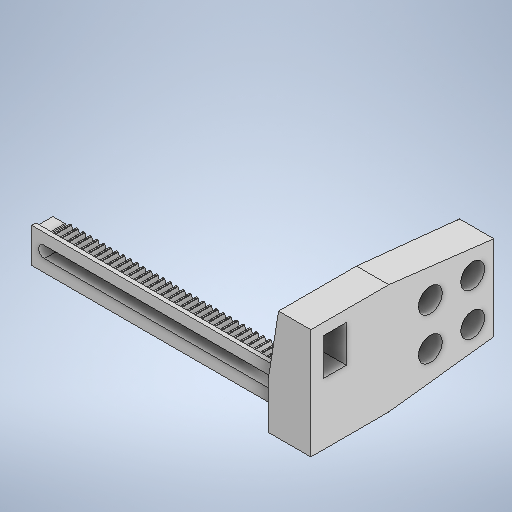
# Autodesk Inventor part: Gripper_Finger
Saved by Autodesk Inventor 2025.1 (Build 291241000, 241)
## iProperties
Created: 2024-08-01
Part Number: Gripper_Finger
Material: Generic
Document SubType Name: Modeling
Designer: leonh
Density: 1 g/cm^3
Appearance: Default
Author: leonh
Autodesk Inventor part; units mm, degrees
(part 1 of 3)
ref_plane "YZ Plane" through (0, 0, 0) normal (1, 0, 0) x (0, 1, 0)
ref_plane "XZ Plane" through (0, 0, 0) normal (0, 1, 0) x (-1, 0, 0)
sketch "Sketch1" plane through (0, 0, 0) normal (0, 0, 1) x (1, 0, 0)
  line L0 (-2.8751, 1.4125) -> (2.9873, 1.4125) construction
  line L1 (-2.8751, 0.2875) -> (2.9873, 0.2875) construction
  line L2 (-2.4544, 1.4586) -> (-2.4544, -0.4067) construction
  line L3 (-2.0617, 1.4586) -> (-2.0617, -0.3717) construction
  line L4 (-1.669, 1.4586) -> (-1.669, -0.4628) construction
  line L5 (-1.2763, 1.4586) -> (-1.2763, -0.4628) construction
  line L6 (-0.8836, 1.4586) -> (-0.8836, -0.5795) construction
  line L7 (-2.8751, 0.9125) -> (-2.5944, 0.9125) construction
  line L8 (-1.8366, 0.452) -> (-1.669, 0.9125)
  line L9 (-1.669, 0.9125) -> (-1.5109, 1.3467)
  line L10 (-1.0416, 1.3467) -> (-0.8836, 0.9125)
  line L11 (-2.2868, 0.452) -> (-2.4065, 0.7809)
  line L12 (-1.417, 1.4125) -> (-1.0656, 1.4125) construction
  line L13 (-2.0518, 0.2875) -> (-2.0715, 0.2875)
  line L14 (-1.487, 1.4125) -> (-1.1356, 1.4125)
  arc A0 (-2.2868, 0.452) -> (-2.0518, 0.2875) centre (-2.0518, 0.5375) ccw
  arc A1 (-2.0715, 0.2875) -> (-1.8366, 0.452) centre (-2.0715, 0.5375) ccw
  arc A2 (-1.417, 1.4125) -> (-1.5109, 1.3467) centre (-1.417, 1.3125) ccw
  arc A3 (-1.0416, 1.3467) -> (-1.1356, 1.4125) centre (-1.1356, 1.3125) ccw
  arc A4 (0.5292, 1.3467) -> (0.4352, 1.4125) centre (0.4352, 1.3125) ccw
  line L15 (0.1538, 1.4125) -> (0.5052, 1.4125) construction
  arc A5 (0.1538, 1.4125) -> (0.0599, 1.3467) centre (0.1538, 1.3125) ccw
  line L16 (-0.0982, 0.9125) -> (0.0599, 1.3467)
  line L17 (0.0838, 1.4125) -> (0.4352, 1.4125)
  line L18 (-0.2658, 0.452) -> (-0.0982, 0.9125)
  arc A6 (-0.5007, 0.2875) -> (-0.2658, 0.452) centre (-0.5007, 0.5375) ccw
  line L19 (-0.481, 0.2875) -> (-0.5007, 0.2875)
  arc A7 (-0.716, 0.452) -> (-0.481, 0.2875) centre (-0.481, 0.5375) ccw
  line L20 (-0.716, 0.452) -> (-0.8836, 0.9125)
  line L21 (0.5292, 1.3467) -> (0.6872, 0.9125)
  arc A8 (2.1, 1.3467) -> (2.006, 1.4125) centre (2.006, 1.3125) ccw
  line L22 (1.7246, 1.4125) -> (2.076, 1.4125) construction
  arc A9 (1.7246, 1.4125) -> (1.6307, 1.3467) centre (1.7246, 1.3125) ccw
  line L23 (1.4726, 0.9125) -> (1.6307, 1.3467)
  line L24 (1.6546, 1.4125) -> (2.006, 1.4125)
  line L25 (1.305, 0.452) -> (1.4726, 0.9125)
  arc A10 (1.0701, 0.2875) -> (1.305, 0.452) centre (1.0701, 0.5375) ccw
  line L26 (1.0898, 0.2875) -> (1.0701, 0.2875)
  arc A11 (0.8548, 0.452) -> (1.0898, 0.2875) centre (1.0898, 0.5375) ccw
  line L27 (0.8548, 0.452) -> (0.6872, 0.9125)
  line L28 (2.1, 1.3467) -> (2.258, 0.9125)
  arc A12 (3.6708, 1.3467) -> (3.5768, 1.4125) centre (3.5768, 1.3125) ccw
  line L29 (3.2954, 1.4125) -> (3.6468, 1.4125) construction
  arc A13 (3.2954, 1.4125) -> (3.2015, 1.3467) centre (3.2954, 1.3125) ccw
  line L30 (3.0434, 0.9125) -> (3.2015, 1.3467)
  line L31 (3.2254, 1.4125) -> (3.5768, 1.4125)
  line L32 (2.8758, 0.452) -> (3.0434, 0.9125)
  arc A14 (2.6409, 0.2875) -> (2.8758, 0.452) centre (2.6409, 0.5375) ccw
  line L33 (2.6606, 0.2875) -> (2.6409, 0.2875)
  arc A15 (2.4256, 0.452) -> (2.6606, 0.2875) centre (2.6606, 0.5375) ccw
  line L34 (2.4256, 0.452) -> (2.258, 0.9125)
  line L35 (3.6708, 1.3467) -> (3.8288, 0.9125)
  arc A16 (5.2416, 1.3467) -> (5.1476, 1.4125) centre (5.1476, 1.3125) ccw
  line L36 (4.8662, 1.4125) -> (5.2176, 1.4125) construction
  arc A17 (4.8662, 1.4125) -> (4.7723, 1.3467) centre (4.8662, 1.3125) ccw
  line L37 (4.6142, 0.9125) -> (4.7723, 1.3467)
  line L38 (4.7962, 1.4125) -> (5.1476, 1.4125)
  line L39 (4.4466, 0.452) -> (4.6142, 0.9125)
  arc A18 (4.2117, 0.2875) -> (4.4466, 0.452) centre (4.2117, 0.5375) ccw
  line L40 (4.2313, 0.2875) -> (4.2117, 0.2875)
  arc A19 (3.9964, 0.452) -> (4.2313, 0.2875) centre (4.2313, 0.5375) ccw
  line L41 (3.9964, 0.452) -> (3.8288, 0.9125)
  line L42 (5.2416, 1.3467) -> (5.3996, 0.9125)
  arc A20 (6.8124, 1.3467) -> (6.7184, 1.4125) centre (6.7184, 1.3125) ccw
  line L43 (6.437, 1.4125) -> (6.7884, 1.4125) construction
  arc A21 (6.437, 1.4125) -> (6.343, 1.3467) centre (6.437, 1.3125) ccw
  line L44 (6.185, 0.9125) -> (6.343, 1.3467)
  line L45 (6.367, 1.4125) -> (6.7184, 1.4125)
  line L46 (6.0174, 0.452) -> (6.185, 0.9125)
  arc A22 (5.7825, 0.2875) -> (6.0174, 0.452) centre (5.7825, 0.5375) ccw
  line L47 (5.8021, 0.2875) -> (5.7825, 0.2875)
  arc A23 (5.5672, 0.452) -> (5.8021, 0.2875) centre (5.8021, 0.5375) ccw
  line L48 (5.5672, 0.452) -> (5.3996, 0.9125)
  line L49 (6.8124, 1.3467) -> (6.9704, 0.9125)
  arc A24 (8.3832, 1.3467) -> (8.2892, 1.4125) centre (8.2892, 1.3125) ccw
  line L50 (8.0078, 1.4125) -> (8.3592, 1.4125) construction
  arc A25 (8.0078, 1.4125) -> (7.9138, 1.3467) centre (8.0078, 1.3125) ccw
  line L51 (7.7558, 0.9125) -> (7.9138, 1.3467)
  line L52 (7.9378, 1.4125) -> (8.2892, 1.4125)
  line L53 (7.5882, 0.452) -> (7.7558, 0.9125)
  arc A26 (7.3533, 0.2875) -> (7.5882, 0.452) centre (7.3533, 0.5375) ccw
  line L54 (7.3729, 0.2875) -> (7.3533, 0.2875)
  arc A27 (7.138, 0.452) -> (7.3729, 0.2875) centre (7.3729, 0.5375) ccw
  line L55 (7.138, 0.452) -> (6.9704, 0.9125)
  line L56 (8.3832, 1.3467) -> (8.5412, 0.9125)
  arc A28 (9.954, 1.3467) -> (9.86, 1.4125) centre (9.86, 1.3125) ccw
  line L57 (9.5786, 1.4125) -> (9.93, 1.4125) construction
  arc A29 (9.5786, 1.4125) -> (9.4846, 1.3467) centre (9.5786, 1.3125) ccw
  line L58 (9.3266, 0.9125) -> (9.4846, 1.3467)
  line L59 (9.5086, 1.4125) -> (9.86, 1.4125)
  line L60 (9.159, 0.452) -> (9.3266, 0.9125)
  arc A30 (8.9241, 0.2875) -> (9.159, 0.452) centre (8.9241, 0.5375) ccw
  line L61 (8.9437, 0.2875) -> (8.9241, 0.2875)
  arc A31 (8.7088, 0.452) -> (8.9437, 0.2875) centre (8.9437, 0.5375) ccw
  line L62 (8.7088, 0.452) -> (8.5412, 0.9125)
  line L63 (9.954, 1.3467) -> (10.112, 0.9125)
  arc A32 (11.5248, 1.3467) -> (11.4308, 1.4125) centre (11.4308, 1.3125) ccw
  line L64 (11.1494, 1.4125) -> (11.5008, 1.4125) construction
  arc A33 (11.1494, 1.4125) -> (11.0554, 1.3467) centre (11.1494, 1.3125) ccw
  line L65 (10.8974, 0.9125) -> (11.0554, 1.3467)
  line L66 (11.0794, 1.4125) -> (11.4308, 1.4125)
  line L67 (10.7298, 0.452) -> (10.8974, 0.9125)
  arc A34 (10.4949, 0.2875) -> (10.7298, 0.452) centre (10.4949, 0.5375) ccw
  line L68 (10.5145, 0.2875) -> (10.4949, 0.2875)
  arc A35 (10.2796, 0.452) -> (10.5145, 0.2875) centre (10.5145, 0.5375) ccw
  line L69 (10.2796, 0.452) -> (10.112, 0.9125)
  line L70 (11.5248, 1.3467) -> (11.6828, 0.9125)
  arc A36 (13.0956, 1.3467) -> (13.0016, 1.4125) centre (13.0016, 1.3125) ccw
  line L71 (12.7202, 1.4125) -> (13.0716, 1.4125) construction
  arc A37 (12.7202, 1.4125) -> (12.6262, 1.3467) centre (12.7202, 1.3125) ccw
  line L72 (12.4682, 0.9125) -> (12.6262, 1.3467)
  line L73 (12.6502, 1.4125) -> (13.0016, 1.4125)
  line L74 (12.3006, 0.452) -> (12.4682, 0.9125)
  arc A38 (12.0657, 0.2875) -> (12.3006, 0.452) centre (12.0657, 0.5375) ccw
  line L75 (12.0853, 0.2875) -> (12.0657, 0.2875)
  arc A39 (11.8504, 0.452) -> (12.0853, 0.2875) centre (12.0853, 0.5375) ccw
  line L76 (11.8504, 0.452) -> (11.6828, 0.9125)
  line L77 (13.0956, 1.3467) -> (13.2536, 0.9125)
  arc A40 (14.6664, 1.3467) -> (14.5724, 1.4125) centre (14.5724, 1.3125) ccw
  line L78 (14.291, 1.4125) -> (14.6424, 1.4125) construction
  arc A41 (14.291, 1.4125) -> (14.197, 1.3467) centre (14.291, 1.3125) ccw
  line L79 (14.039, 0.9125) -> (14.197, 1.3467)
  line L80 (14.221, 1.4125) -> (14.5724, 1.4125)
  line L81 (13.8714, 0.452) -> (14.039, 0.9125)
  arc A42 (13.6365, 0.2875) -> (13.8714, 0.452) centre (13.6365, 0.5375) ccw
  line L82 (13.6561, 0.2875) -> (13.6365, 0.2875)
  arc A43 (13.4212, 0.452) -> (13.6561, 0.2875) centre (13.6561, 0.5375) ccw
  line L83 (13.4212, 0.452) -> (13.2536, 0.9125)
  line L84 (14.6664, 1.3467) -> (14.8244, 0.9125)
  arc A44 (16.2372, 1.3467) -> (16.1432, 1.4125) centre (16.1432, 1.3125) ccw
  line L85 (15.8618, 1.4125) -> (16.2132, 1.4125) construction
  arc A45 (15.8618, 1.4125) -> (15.7678, 1.3467) centre (15.8618, 1.3125) ccw
  line L86 (15.6098, 0.9125) -> (15.7678, 1.3467)
  line L87 (15.7918, 1.4125) -> (16.1432, 1.4125)
  line L88 (15.4422, 0.452) -> (15.6098, 0.9125)
  arc A46 (15.2073, 0.2875) -> (15.4422, 0.452) centre (15.2073, 0.5375) ccw
  line L89 (15.2269, 0.2875) -> (15.2073, 0.2875)
  arc A47 (14.992, 0.452) -> (15.2269, 0.2875) centre (15.2269, 0.5375) ccw
  line L90 (14.992, 0.452) -> (14.8244, 0.9125)
  line L91 (16.2372, 1.3467) -> (16.3952, 0.9125)
  arc A48 (17.8079, 1.3467) -> (17.714, 1.4125) centre (17.714, 1.3125) ccw
  line L92 (17.4326, 1.4125) -> (17.784, 1.4125) construction
  arc A49 (17.4326, 1.4125) -> (17.3386, 1.3467) centre (17.4326, 1.3125) ccw
  line L93 (17.1806, 0.9125) -> (17.3386, 1.3467)
  line L94 (17.3626, 1.4125) -> (17.714, 1.4125)
  line L95 (17.013, 0.452) -> (17.1806, 0.9125)
  arc A50 (16.7781, 0.2875) -> (17.013, 0.452) centre (16.7781, 0.5375) ccw
  line L96 (16.7977, 0.2875) -> (16.7781, 0.2875)
  arc A51 (16.5628, 0.452) -> (16.7977, 0.2875) centre (16.7977, 0.5375) ccw
  line L97 (16.5628, 0.452) -> (16.3952, 0.9125)
  line L98 (17.8079, 1.3467) -> (17.966, 0.9125)
  arc A52 (19.3787, 1.3467) -> (19.2848, 1.4125) centre (19.2848, 1.3125) ccw
  line L99 (19.0034, 1.4125) -> (19.3548, 1.4125) construction
  arc A53 (19.0034, 1.4125) -> (18.9094, 1.3467) centre (19.0034, 1.3125) ccw
  line L100 (18.7514, 0.9125) -> (18.9094, 1.3467)
  line L101 (18.9334, 1.4125) -> (19.2848, 1.4125)
  line L102 (18.5838, 0.452) -> (18.7514, 0.9125)
  arc A54 (18.3488, 0.2875) -> (18.5838, 0.452) centre (18.3488, 0.5375) ccw
  line L103 (18.3685, 0.2875) -> (18.3488, 0.2875)
  arc A55 (18.1336, 0.452) -> (18.3685, 0.2875) centre (18.3685, 0.5375) ccw
  line L104 (18.1336, 0.452) -> (17.966, 0.9125)
  line L105 (19.3787, 1.3467) -> (19.5368, 0.9125)
  arc A56 (20.9495, 1.3467) -> (20.8556, 1.4125) centre (20.8556, 1.3125) ccw
  line L106 (20.5742, 1.4125) -> (20.9256, 1.4125) construction
  arc A57 (20.5742, 1.4125) -> (20.4802, 1.3467) centre (20.5742, 1.3125) ccw
  line L107 (20.3222, 0.9125) -> (20.4802, 1.3467)
  line L108 (20.5042, 1.4125) -> (20.8556, 1.4125)
  line L109 (20.1546, 0.452) -> (20.3222, 0.9125)
  arc A58 (19.9196, 0.2875) -> (20.1546, 0.452) centre (19.9196, 0.5375) ccw
  line L110 (19.9393, 0.2875) -> (19.9196, 0.2875)
  arc A59 (19.7044, 0.452) -> (19.9393, 0.2875) centre (19.9393, 0.5375) ccw
  line L111 (19.7044, 0.452) -> (19.5368, 0.9125)
  line L112 (20.9495, 1.3467) -> (21.1076, 0.9125)
  arc A60 (22.5203, 1.3467) -> (22.4264, 1.4125) centre (22.4264, 1.3125) ccw
  line L113 (22.145, 1.4125) -> (22.4964, 1.4125) construction
  arc A61 (22.145, 1.4125) -> (22.051, 1.3467) centre (22.145, 1.3125) ccw
  line L114 (21.893, 0.9125) -> (22.051, 1.3467)
  line L115 (22.075, 1.4125) -> (22.4264, 1.4125)
  line L116 (21.7254, 0.452) -> (21.893, 0.9125)
  arc A62 (21.4904, 0.2875) -> (21.7254, 0.452) centre (21.4904, 0.5375) ccw
  line L117 (21.5101, 0.2875) -> (21.4904, 0.2875)
  arc A63 (21.2752, 0.452) -> (21.5101, 0.2875) centre (21.5101, 0.5375) ccw
  line L118 (21.2752, 0.452) -> (21.1076, 0.9125)
  line L119 (22.5203, 1.3467) -> (22.6784, 0.9125)
  arc A64 (24.0911, 1.3467) -> (23.9972, 1.4125) centre (23.9972, 1.3125) ccw
  line L120 (23.7158, 1.4125) -> (24.0672, 1.4125) construction
  arc A65 (23.7158, 1.4125) -> (23.6218, 1.3467) centre (23.7158, 1.3125) ccw
  line L121 (23.4638, 0.9125) -> (23.6218, 1.3467)
  line L122 (23.6458, 1.4125) -> (23.9972, 1.4125)
  line L123 (23.2962, 0.452) -> (23.4638, 0.9125)
  arc A66 (23.0612, 0.2875) -> (23.2962, 0.452) centre (23.0612, 0.5375) ccw
  line L124 (23.0809, 0.2875) -> (23.0612, 0.2875)
  arc A67 (22.846, 0.452) -> (23.0809, 0.2875) centre (23.0809, 0.5375) ccw
  line L125 (22.846, 0.452) -> (22.6784, 0.9125)
  line L126 (24.0911, 1.3467) -> (24.2492, 0.9125)
  arc A68 (25.6619, 1.3467) -> (25.568, 1.4125) centre (25.568, 1.3125) ccw
  line L127 (25.2866, 1.4125) -> (25.638, 1.4125) construction
  arc A69 (25.2866, 1.4125) -> (25.1926, 1.3467) centre (25.2866, 1.3125) ccw
  line L128 (25.0346, 0.9125) -> (25.1926, 1.3467)
  line L129 (25.2166, 1.4125) -> (25.568, 1.4125)
  line L130 (24.867, 0.452) -> (25.0346, 0.9125)
  arc A70 (24.632, 0.2875) -> (24.867, 0.452) centre (24.632, 0.5375) ccw
  line L131 (24.6517, 0.2875) -> (24.632, 0.2875)
  arc A71 (24.4168, 0.452) -> (24.6517, 0.2875) centre (24.6517, 0.5375) ccw
  line L132 (24.4168, 0.452) -> (24.2492, 0.9125)
  line L133 (25.6619, 1.3467) -> (25.82, 0.9125)
  arc A72 (27.2327, 1.3467) -> (27.1388, 1.4125) centre (27.1388, 1.3125) ccw
  line L134 (26.8574, 1.4125) -> (27.2088, 1.4125) construction
  arc A73 (26.8574, 1.4125) -> (26.7634, 1.3467) centre (26.8574, 1.3125) ccw
  line L135 (26.6054, 0.9125) -> (26.7634, 1.3467)
  line L136 (26.7873, 1.4125) -> (27.1388, 1.4125)
  line L137 (26.4378, 0.452) -> (26.6054, 0.9125)
  arc A74 (26.2028, 0.2875) -> (26.4378, 0.452) centre (26.2028, 0.5375) ccw
  line L138 (26.2225, 0.2875) -> (26.2028, 0.2875)
  arc A75 (25.9876, 0.452) -> (26.2225, 0.2875) centre (26.2225, 0.5375) ccw
  line L139 (25.9876, 0.452) -> (25.82, 0.9125)
  line L140 (27.2327, 1.3467) -> (27.3908, 0.9125)
  arc A76 (28.8035, 1.3467) -> (28.7096, 1.4125) centre (28.7096, 1.3125) ccw
  line L141 (28.4282, 1.4125) -> (28.7796, 1.4125) construction
  arc A77 (28.4282, 1.4125) -> (28.3342, 1.3467) centre (28.4282, 1.3125) ccw
  line L142 (28.1762, 0.9125) -> (28.3342, 1.3467)
  line L143 (28.3581, 1.4125) -> (28.7096, 1.4125)
  line L144 (28.0085, 0.452) -> (28.1762, 0.9125)
  arc A78 (27.7736, 0.2875) -> (28.0085, 0.452) centre (27.7736, 0.5375) ccw
  line L145 (27.7933, 0.2875) -> (27.7736, 0.2875)
  arc A79 (27.5584, 0.452) -> (27.7933, 0.2875) centre (27.7933, 0.5375) ccw
  line L146 (27.5584, 0.452) -> (27.3908, 0.9125)
  line L147 (28.8035, 1.3467) -> (28.9616, 0.9125)
  arc A80 (30.3743, 1.3467) -> (30.2803, 1.4125) centre (30.2803, 1.3125) ccw
  line L148 (29.999, 1.4125) -> (30.3504, 1.4125) construction
  arc A81 (29.999, 1.4125) -> (29.905, 1.3467) centre (29.999, 1.3125) ccw
  line L149 (29.747, 0.9125) -> (29.905, 1.3467)
  line L150 (29.9289, 1.4125) -> (30.2803, 1.4125)
  line L151 (29.5793, 0.452) -> (29.747, 0.9125)
  arc A82 (29.3444, 0.2875) -> (29.5793, 0.452) centre (29.3444, 0.5375) ccw
  line L152 (29.3641, 0.2875) -> (29.3444, 0.2875)
  arc A83 (29.1292, 0.452) -> (29.3641, 0.2875) centre (29.3641, 0.5375) ccw
  line L153 (29.1292, 0.452) -> (28.9616, 0.9125)
  line L154 (30.3743, 1.3467) -> (30.5324, 0.9125)
  arc A84 (31.9451, 1.3467) -> (31.8511, 1.4125) centre (31.8511, 1.3125) ccw
  line L155 (31.5698, 1.4125) -> (31.9212, 1.4125) construction
  arc A85 (31.5698, 1.4125) -> (31.4758, 1.3467) centre (31.5698, 1.3125) ccw
  line L156 (31.3178, 0.9125) -> (31.4758, 1.3467)
  line L157 (31.4997, 1.4125) -> (31.8511, 1.4125)
  line L158 (31.1501, 0.452) -> (31.3178, 0.9125)
  arc A86 (30.9152, 0.2875) -> (31.1501, 0.452) centre (30.9152, 0.5375) ccw
  line L159 (30.9349, 0.2875) -> (30.9152, 0.2875)
  arc A87 (30.7, 0.452) -> (30.9349, 0.2875) centre (30.9349, 0.5375) ccw
  line L160 (30.7, 0.452) -> (30.5324, 0.9125)
  line L161 (31.9451, 1.3467) -> (32.1031, 0.9125)
  arc A88 (33.5159, 1.3467) -> (33.4219, 1.4125) centre (33.4219, 1.3125) ccw
  line L162 (33.1406, 1.4125) -> (33.492, 1.4125) construction
  arc A89 (33.1406, 1.4125) -> (33.0466, 1.3467) centre (33.1406, 1.3125) ccw
  line L163 (32.8885, 0.9125) -> (33.0466, 1.3467)
  line L164 (33.0705, 1.4125) -> (33.4219, 1.4125)
  line L165 (32.7209, 0.452) -> (32.8885, 0.9125)
  arc A90 (32.486, 0.2875) -> (32.7209, 0.452) centre (32.486, 0.5375) ccw
  line L166 (32.5057, 0.2875) -> (32.486, 0.2875)
  arc A91 (32.2708, 0.452) -> (32.5057, 0.2875) centre (32.5057, 0.5375) ccw
  line L167 (32.2708, 0.452) -> (32.1031, 0.9125)
  line L168 (33.5159, 1.3467) -> (33.6739, 0.9125)
  arc A92 (35.0867, 1.3467) -> (34.9927, 1.4125) centre (34.9927, 1.3125) ccw
  line L169 (34.7114, 1.4125) -> (35.0628, 1.4125) construction
  arc A93 (34.7114, 1.4125) -> (34.6174, 1.3467) centre (34.7114, 1.3125) ccw
  line L170 (34.4593, 0.9125) -> (34.6174, 1.3467)
  line L171 (34.6413, 1.4125) -> (34.9927, 1.4125)
  line L172 (34.2917, 0.452) -> (34.4593, 0.9125)
  arc A94 (34.0568, 0.2875) -> (34.2917, 0.452) centre (34.0568, 0.5375) ccw
  line L173 (34.0765, 0.2875) -> (34.0568, 0.2875)
  arc A95 (33.8416, 0.452) -> (34.0765, 0.2875) centre (34.0765, 0.5375) ccw
  line L174 (33.8416, 0.452) -> (33.6739, 0.9125)
  line L175 (35.0867, 1.3467) -> (35.2447, 0.9125)
  arc A96 (36.6575, 1.3467) -> (36.5635, 1.4125) centre (36.5635, 1.3125) ccw
  line L176 (36.2821, 1.4125) -> (36.6336, 1.4125) construction
  arc A97 (36.2821, 1.4125) -> (36.1882, 1.3467) centre (36.2821, 1.3125) ccw
  line L177 (36.0301, 0.9125) -> (36.1882, 1.3467)
  line L178 (36.2121, 1.4125) -> (36.5635, 1.4125)
  line L179 (35.8625, 0.452) -> (36.0301, 0.9125)
  arc A98 (35.6276, 0.2875) -> (35.8625, 0.452) centre (35.6276, 0.5375) ccw
  line L180 (35.6473, 0.2875) -> (35.6276, 0.2875)
  arc A99 (35.4124, 0.452) -> (35.6473, 0.2875) centre (35.6473, 0.5375) ccw
  line L181 (35.4124, 0.452) -> (35.2447, 0.9125)
  line L182 (36.6575, 1.3467) -> (36.8155, 0.9125)
  arc A100 (38.2283, 1.3467) -> (38.1343, 1.4125) centre (38.1343, 1.3125) ccw
  line L183 (37.8529, 1.4125) -> (38.2044, 1.4125) construction
  arc A101 (37.8529, 1.4125) -> (37.759, 1.3467) centre (37.8529, 1.3125) ccw
  line L184 (37.6009, 0.9125) -> (37.759, 1.3467)
  line L185 (37.7829, 1.4125) -> (38.1343, 1.4125)
  line L186 (37.4333, 0.452) -> (37.6009, 0.9125)
  arc A102 (37.1984, 0.2875) -> (37.4333, 0.452) centre (37.1984, 0.5375) ccw
  line L187 (37.2181, 0.2875) -> (37.1984, 0.2875)
  arc A103 (36.9831, 0.452) -> (37.2181, 0.2875) centre (37.2181, 0.5375) ccw
  line L188 (36.9831, 0.452) -> (36.8155, 0.9125)
  line L189 (38.2283, 1.3467) -> (38.3863, 0.9125)
  arc A104 (39.7991, 1.3467) -> (39.7051, 1.4125) centre (39.7051, 1.3125) ccw
  line L190 (39.4237, 1.4125) -> (39.7751, 1.4125) construction
  arc A105 (39.4237, 1.4125) -> (39.3298, 1.3467) centre (39.4237, 1.3125) ccw
  line L191 (39.1717, 0.9125) -> (39.3298, 1.3467)
  line L192 (39.3537, 1.4125) -> (39.7051, 1.4125)
  line L193 (39.0041, 0.452) -> (39.1717, 0.9125)
  arc A106 (38.7692, 0.2875) -> (39.0041, 0.452) centre (38.7692, 0.5375) ccw
  line L194 (38.7889, 0.2875) -> (38.7692, 0.2875)
  arc A107 (38.5539, 0.452) -> (38.7889, 0.2875) centre (38.7889, 0.5375) ccw
  line L195 (38.5539, 0.452) -> (38.3863, 0.9125)
  line L196 (39.7991, 1.3467) -> (39.9571, 0.9125)
  arc A108 (41.3699, 1.3467) -> (41.2759, 1.4125) centre (41.2759, 1.3125) ccw
  line L197 (40.9945, 1.4125) -> (41.3459, 1.4125) construction
  arc A109 (40.9945, 1.4125) -> (40.9006, 1.3467) centre (40.9945, 1.3125) ccw
  line L198 (40.7425, 0.9125) -> (40.9006, 1.3467)
  line L199 (40.9245, 1.4125) -> (41.2759, 1.4125)
  line L200 (40.5749, 0.452) -> (40.7425, 0.9125)
  arc A110 (40.34, 0.2875) -> (40.5749, 0.452) centre (40.34, 0.5375) ccw
  line L201 (40.3597, 0.2875) -> (40.34, 0.2875)
  arc A111 (40.1247, 0.452) -> (40.3597, 0.2875) centre (40.3597, 0.5375) ccw
  line L202 (40.1247, 0.452) -> (39.9571, 0.9125)
  line L203 (41.3699, 1.3467) -> (41.5279, 0.9125)
  arc A112 (42.9407, 1.3467) -> (42.8467, 1.4125) centre (42.8467, 1.3125) ccw
  line L204 (42.5653, 1.4125) -> (42.9167, 1.4125) construction
  arc A113 (42.5653, 1.4125) -> (42.4714, 1.3467) centre (42.5653, 1.3125) ccw
  line L205 (42.3133, 0.9125) -> (42.4714, 1.3467)
  line L206 (42.4953, 1.4125) -> (42.8467, 1.4125)
  line L207 (42.1457, 0.452) -> (42.3133, 0.9125)
  arc A114 (41.9108, 0.2875) -> (42.1457, 0.452) centre (41.9108, 0.5375) ccw
  line L208 (41.9305, 0.2875) -> (41.9108, 0.2875)
  arc A115 (41.6955, 0.452) -> (41.9305, 0.2875) centre (41.9305, 0.5375) ccw
  line L209 (41.6955, 0.452) -> (41.5279, 0.9125)
  line L210 (42.9407, 1.3467) -> (43.0987, 0.9125)
  arc A116 (44.5115, 1.3467) -> (44.4175, 1.4125) centre (44.4175, 1.3125) ccw
  line L211 (44.1361, 1.4125) -> (44.4875, 1.4125) construction
  arc A117 (44.1361, 1.4125) -> (44.0422, 1.3467) centre (44.1361, 1.3125) ccw
  line L212 (43.8841, 0.9125) -> (44.0422, 1.3467)
  line L213 (44.0661, 1.4125) -> (44.4175, 1.4125)
  line L214 (43.7165, 0.452) -> (43.8841, 0.9125)
  arc A118 (43.4816, 0.2875) -> (43.7165, 0.452) centre (43.4816, 0.5375) ccw
  line L215 (43.5013, 0.2875) -> (43.4816, 0.2875)
  arc A119 (43.2663, 0.452) -> (43.5013, 0.2875) centre (43.5013, 0.5375) ccw
  line L216 (43.2663, 0.452) -> (43.0987, 0.9125)
  line L217 (44.5115, 1.3467) -> (44.6695, 0.9125)
  arc A120 (46.0823, 1.3467) -> (45.9883, 1.4125) centre (45.9883, 1.3125) ccw
  line L218 (45.7069, 1.4125) -> (46.0583, 1.4125) construction
  arc A121 (45.7069, 1.4125) -> (45.613, 1.3467) centre (45.7069, 1.3125) ccw
  line L219 (45.4549, 0.9125) -> (45.613, 1.3467)
  line L220 (45.6369, 1.4125) -> (45.9883, 1.4125)
  line L221 (45.2873, 0.452) -> (45.4549, 0.9125)
  arc A122 (45.0524, 0.2875) -> (45.2873, 0.452) centre (45.0524, 0.5375) ccw
  line L222 (45.0721, 0.2875) -> (45.0524, 0.2875)
  arc A123 (44.8371, 0.452) -> (45.0721, 0.2875) centre (45.0721, 0.5375) ccw
  line L223 (44.8371, 0.452) -> (44.6695, 0.9125)
  line L224 (46.0823, 1.3467) -> (46.2403, 0.9125)
  arc A124 (47.6531, 1.3467) -> (47.5591, 1.4125) centre (47.5591, 1.3125) ccw
  line L225 (47.2777, 1.4125) -> (47.6291, 1.4125) construction
  arc A125 (47.2777, 1.4125) -> (47.1838, 1.3467) centre (47.2777, 1.3125) ccw
  line L226 (47.0257, 0.9125) -> (47.1838, 1.3467)
  line L227 (47.2077, 1.4125) -> (47.5591, 1.4125)
  line L228 (46.8581, 0.452) -> (47.0257, 0.9125)
  arc A126 (46.6232, 0.2875) -> (46.8581, 0.452) centre (46.6232, 0.5375) ccw
  line L229 (46.6429, 0.2875) -> (46.6232, 0.2875)
  arc A127 (46.4079, 0.452) -> (46.6429, 0.2875) centre (46.6429, 0.5375) ccw
  line L230 (46.4079, 0.452) -> (46.2403, 0.9125)
  line L231 (47.6531, 1.3467) -> (47.8111, 0.9125)
  arc A128 (49.2239, 1.3467) -> (49.1299, 1.4125) centre (49.1299, 1.3125) ccw
  line L232 (48.8485, 1.4125) -> (49.1999, 1.4125) construction
  arc A129 (48.8485, 1.4125) -> (48.7545, 1.3467) centre (48.8485, 1.3125) ccw
  line L233 (48.5965, 0.9125) -> (48.7545, 1.3467)
  line L234 (48.7785, 1.4125) -> (49.1299, 1.4125)
  line L235 (48.4289, 0.452) -> (48.5965, 0.9125)
  arc A130 (48.194, 0.2875) -> (48.4289, 0.452) centre (48.194, 0.5375) ccw
  line L236 (48.2136, 0.2875) -> (48.194, 0.2875)
  arc A131 (47.9787, 0.452) -> (48.2136, 0.2875) centre (48.2136, 0.5375) ccw
  line L237 (47.9787, 0.452) -> (47.8111, 0.9125)
  line L238 (49.2239, 1.3467) -> (49.3819, 0.9125)
  arc A132 (50.7947, 1.3467) -> (50.7007, 1.4125) centre (50.7007, 1.3125) ccw
  line L239 (50.4193, 1.4125) -> (50.7707, 1.4125) construction
  arc A133 (50.4193, 1.4125) -> (50.3253, 1.3467) centre (50.4193, 1.3125) ccw
  line L240 (50.1673, 0.9125) -> (50.3253, 1.3467)
  line L241 (50.3493, 1.4125) -> (50.7007, 1.4125)
  line L242 (49.9997, 0.452) -> (50.1673, 0.9125)
  arc A134 (49.7648, 0.2875) -> (49.9997, 0.452) centre (49.7648, 0.5375) ccw
  line L243 (49.7844, 0.2875) -> (49.7648, 0.2875)
  arc A135 (49.5495, 0.452) -> (49.7844, 0.2875) centre (49.7844, 0.5375) ccw
  line L244 (49.5495, 0.452) -> (49.3819, 0.9125)
  line L245 (50.7947, 1.3467) -> (50.9527, 0.9125)
  arc A136 (52.3655, 1.3467) -> (52.2715, 1.4125) centre (52.2715, 1.3125) ccw
  line L246 (51.9901, 1.4125) -> (52.3415, 1.4125) construction
  arc A137 (51.9901, 1.4125) -> (51.8961, 1.3467) centre (51.9901, 1.3125) ccw
  line L247 (51.7381, 0.9125) -> (51.8961, 1.3467)
  line L248 (51.9201, 1.4125) -> (52.2715, 1.4125)
  line L249 (51.5705, 0.452) -> (51.7381, 0.9125)
  arc A138 (51.3356, 0.2875) -> (51.5705, 0.452) centre (51.3356, 0.5375) ccw
  line L250 (51.3552, 0.2875) -> (51.3356, 0.2875)
  arc A139 (51.1203, 0.452) -> (51.3552, 0.2875) centre (51.3552, 0.5375) ccw
  line L251 (51.1203, 0.452) -> (50.9527, 0.9125)
  line L252 (52.3655, 1.3467) -> (52.4756, 1.0441)
  line L253 (-2.4544, 0.9125) -> (-5.4544, 0.9125)
  line L254 (-5.4544, 0.9125) -> (-5.4544, -6.5875)
  line L255 (-5.4544, -6.5875) -> (55.5235, -6.5875)
  line L256 (55.5235, -6.5875) -> (55.5235, 0.9125)
  line L257 (55.5235, 0.9125) -> (52.6635, 0.9125)
  arc A140 (-2.4065, 0.7809) -> (-2.5944, 0.9125) centre (-2.5944, 0.7125) ccw
  arc A141 (52.4756, 1.0441) -> (52.6635, 0.9125) centre (52.6635, 1.1125) ccw
  point P0 (0, 0)
  point P1 (-1.8965, 0.2875)
  point P2 (-2.2269, 0.2875)
  point P3 (0.6872, 1.4586)
  point P4 (0.2945, 1.4586)
  point P5 (-0.4909, 1.4586)
  point P6 (-0.8836, 1.4586)
  point P7 (-0.0982, 1.4586)
  point P8 (-0.3257, 0.2875)
  point P9 (-0.6561, 0.2875)
  point P10 (2.258, 1.4586)
  point P11 (1.8653, 1.4586)
  point P12 (1.0799, 1.4586)
  point P13 (0.6872, 1.4586)
  point P14 (1.4726, 1.4586)
  point P15 (1.2451, 0.2875)
  point P16 (0.9147, 0.2875)
  point P17 (3.8288, 1.4586)
  point P18 (3.4361, 1.4586)
  point P19 (2.6507, 1.4586)
  point P20 (2.258, 1.4586)
  point P21 (3.0434, 1.4586)
  point P22 (2.8159, 0.2875)
  point P23 (2.4855, 0.2875)
  point P24 (5.3996, 1.4586)
  point P25 (5.0069, 1.4586)
  point P26 (4.2215, 1.4586)
  point P27 (3.8288, 1.4586)
  point P28 (4.6142, 1.4586)
  point P29 (4.3867, 0.2875)
  point P30 (4.0563, 0.2875)
  point P31 (6.9704, 1.4586)
  point P32 (6.5777, 1.4586)
  point P33 (5.7923, 1.4586)
  point P34 (5.3996, 1.4586)
  point P35 (6.185, 1.4586)
  point P36 (5.9575, 0.2875)
  point P37 (5.6271, 0.2875)
  point P38 (8.5412, 1.4586)
  point P39 (8.1485, 1.4586)
  point P40 (7.3631, 1.4586)
  point P41 (6.9704, 1.4586)
  point P42 (7.7558, 1.4586)
  point P43 (7.5283, 0.2875)
  point P44 (7.1979, 0.2875)
  point P45 (10.112, 1.4586)
  point P46 (9.7193, 1.4586)
  point P47 (8.9339, 1.4586)
  point P48 (8.5412, 1.4586)
  point P49 (9.3266, 1.4586)
  point P50 (9.0991, 0.2875)
  point P51 (8.7687, 0.2875)
  point P52 (11.6828, 1.4586)
  point P53 (11.2901, 1.4586)
  point P54 (10.5047, 1.4586)
  point P55 (10.112, 1.4586)
  point P56 (10.8974, 1.4586)
  point P57 (10.6699, 0.2875)
  point P58 (10.3395, 0.2875)
  point P59 (13.2536, 1.4586)
  point P60 (12.8609, 1.4586)
  point P61 (12.0755, 1.4586)
  point P62 (11.6828, 1.4586)
  point P63 (12.4682, 1.4586)
  point P64 (12.2407, 0.2875)
  point P65 (11.9103, 0.2875)
  point P66 (14.8244, 1.4586)
  point P67 (14.4317, 1.4586)
  point P68 (13.6463, 1.4586)
  point P69 (13.2536, 1.4586)
  point P70 (14.039, 1.4586)
  point P71 (13.8115, 0.2875)
  point P72 (13.4811, 0.2875)
  point P73 (16.3952, 1.4586)
  point P74 (16.0025, 1.4586)
  point P75 (15.2171, 1.4586)
  point P76 (14.8244, 1.4586)
  point P77 (15.6098, 1.4586)
  point P78 (15.3823, 0.2875)
  point P79 (15.0519, 0.2875)
  point P80 (17.966, 1.4586)
  point P81 (17.5733, 1.4586)
  point P82 (16.7879, 1.4586)
  point P83 (16.3952, 1.4586)
  point P84 (17.1806, 1.4586)
  point P85 (16.9531, 0.2875)
  point P86 (16.6227, 0.2875)
  point P87 (19.5368, 1.4586)
  point P88 (19.1441, 1.4586)
  point P89 (18.3587, 1.4586)
  point P90 (17.966, 1.4586)
  point P91 (18.7514, 1.4586)
  point P92 (18.5239, 0.2875)
  point P93 (18.1935, 0.2875)
  point P94 (21.1076, 1.4586)
  point P95 (20.7149, 1.4586)
  point P96 (19.9295, 1.4586)
  point P97 (19.5368, 1.4586)
  point P98 (20.3222, 1.4586)
  point P99 (20.0947, 0.2875)
  point P100 (19.7643, 0.2875)
  point P101 (22.6784, 1.4586)
  point P102 (22.2857, 1.4586)
  point P103 (21.5003, 1.4586)
  point P104 (21.1076, 1.4586)
  point P105 (21.893, 1.4586)
  point P106 (21.6655, 0.2875)
  point P107 (21.3351, 0.2875)
  point P108 (24.2492, 1.4586)
  point P109 (23.8565, 1.4586)
  point P110 (23.0711, 1.4586)
  point P111 (22.6784, 1.4586)
  point P112 (23.4638, 1.4586)
  point P113 (23.2363, 0.2875)
  point P114 (22.9059, 0.2875)
  point P115 (25.82, 1.4586)
  point P116 (25.4273, 1.4586)
  point P117 (24.6419, 1.4586)
  point P118 (24.2492, 1.4586)
  point P119 (25.0346, 1.4586)
  point P120 (24.8071, 0.2875)
  point P121 (24.4766, 0.2875)
  point P122 (27.3908, 1.4586)
  point P123 (26.9981, 1.4586)
  point P124 (26.2127, 1.4586)
  point P125 (25.82, 1.4586)
  point P126 (26.6054, 1.4586)
  point P127 (26.3779, 0.2875)
  point P128 (26.0474, 0.2875)
  point P129 (28.9616, 1.4586)
  point P130 (28.5689, 1.4586)
  point P131 (27.7835, 1.4586)
  point P132 (27.3908, 1.4586)
  point P133 (28.1762, 1.4586)
  point P134 (27.9487, 0.2875)
  point P135 (27.6182, 0.2875)
  point P136 (30.5324, 1.4586)
  point P137 (30.1397, 1.4586)
  point P138 (29.3543, 1.4586)
  point P139 (28.9616, 1.4586)
  point P140 (29.747, 1.4586)
  point P141 (29.5195, 0.2875)
  point P142 (29.189, 0.2875)
  point P143 (32.1031, 1.4586)
  point P144 (31.7105, 1.4586)
  point P145 (30.9251, 1.4586)
  point P146 (30.5324, 1.4586)
  point P147 (31.3178, 1.4586)
  point P148 (31.0903, 0.2875)
  point P149 (30.7598, 0.2875)
  point P150 (33.6739, 1.4586)
  point P151 (33.2812, 1.4586)
  point P152 (32.4958, 1.4586)
  point P153 (32.1031, 1.4586)
  point P154 (32.8885, 1.4586)
  point P155 (32.6611, 0.2875)
  point P156 (32.3306, 0.2875)
  point P157 (35.2447, 1.4586)
  point P158 (34.852, 1.4586)
  point P159 (34.0666, 1.4586)
  point P160 (33.6739, 1.4586)
  point P161 (34.4593, 1.4586)
  point P162 (34.2319, 0.2875)
  point P163 (33.9014, 0.2875)
  point P164 (36.8155, 1.4586)
  point P165 (36.4228, 1.4586)
  point P166 (35.6374, 1.4586)
  point P167 (35.2447, 1.4586)
  point P168 (36.0301, 1.4586)
  point P169 (35.8027, 0.2875)
  point P170 (35.4722, 0.2875)
  point P171 (38.3863, 1.4586)
  point P172 (37.9936, 1.4586)
  point P173 (37.2082, 1.4586)
  point P174 (36.8155, 1.4586)
  point P175 (37.6009, 1.4586)
  point P176 (37.3735, 0.2875)
  point P177 (37.043, 0.2875)
  point P178 (39.9571, 1.4586)
  point P179 (39.5644, 1.4586)
  point P180 (38.779, 1.4586)
  point P181 (38.3863, 1.4586)
  point P182 (39.1717, 1.4586)
  point P183 (38.9443, 0.2875)
  point P184 (38.6138, 0.2875)
  point P185 (41.5279, 1.4586)
  point P186 (41.1352, 1.4586)
  point P187 (40.3498, 1.4586)
  point P188 (39.9571, 1.4586)
  point P189 (40.7425, 1.4586)
  point P190 (40.515, 0.2875)
  point P191 (40.1846, 0.2875)
  point P192 (43.0987, 1.4586)
  point P193 (42.706, 1.4586)
  point P194 (41.9206, 1.4586)
  point P195 (41.5279, 1.4586)
  point P196 (42.3133, 1.4586)
  point P197 (42.0858, 0.2875)
  point P198 (41.7554, 0.2875)
  point P199 (44.6695, 1.4586)
  dimension "d1" = 0.7854
  dimension "d2" = 0.7854
  dimension "d3" = 1.5708
  dimension "d4" = 1.125
  dimension "d5" = 0.5
  dimension "d6" = 70
  dimension "d7" = 0.25
  dimension "d8" = 0.1
  dimension "d11" = 1.5708
  dimension "d16" = 3
  dimension "d17" = 3
  dimension "d20" = 60.9779
  dimension "d21" = 0.2
  dimension "d41" = 7.5
  constraints: 516 end point, 329 point on line, 284 point on circle, 142 centre point, 12 tangent, 5 horizontal, 5 vertical, 4 perpendicular, 3 collinear, 3 equal radius, 3 midpoint, 1194 other
  measures "d1" distance between parallel lines of L4 L2
  measures "d2" distance between parallel lines of L6 L4
  measures "d3" distance between parallel lines of L6 L2
  measures "d4" distance between parallel lines of L1 L0
  measures "d5" distance between parallel lines of L0 L7
  measures "d6" angle of L0 L9
  measures "d7" radius of A0
  measures "d8" radius of A2
  measures "d11" distance of L10.end L21.end
  measures "d16" distance from line of L253.start L254
  measures "d17" distance from line of L256 point (52.524, 0.913)
  measures "d20" distance of point (55.524, -2.837) point (-5.454, -2.837)
  measures "d21" radius of A140
  measures "d41" distance between parallel lines of L255 L257
extrude "Extrusion1" add sketch "Sketch1" along normal blind 5
sketch "Sketch2" plane through (55.5235, -6.5875, 0) normal (1, 0, 0) x (0, 0, -1)
  line L0 (0, 0) -> (0, 7.5)
  line L1 (0, 7.5) -> (-5, 7.5)
  line L2 (-5, 0) -> (-5, 7.5)
  line L3 (0, 0) -> (-5, 0)
  line L4 (-5, 0) -> (35, 0)
  line L5 (35, 0) -> (35, 20)
  line L6 (35, 20) -> (-5, 20)
  line L7 (-5, 20) -> (-5, 0)
  circle A0 centre (30, 15) radius 2.8
  circle A1 centre (20, 15) radius 2.8
  circle A2 centre (30, 5) radius 2.8
  circle A3 centre (20, 5) radius 2.8
  point P0 (0, 6.5875)
  point P1 (20, 15)
  point P2 (20, 5)
  dimension "d24" = 40
  dimension "d25" = 20
  dimension "d26" = 10
  dimension "d27" = 5
  dimension "d28" = 10
  dimension "d29" = 5
  dimension "d30" = 5.6
  dimension "d33" = 10
  dimension "d36" = 10
  constraints: 8 end point, 4 centre point, 2 horizontal, 2 horizontal alignment, 2 parallel, 2 vertical alignment, 1 coincident, 1 perpendicular, 1 vertical, 6 other
  measures "d24" distance between parallel lines of L5 L7
  measures "d25" distance between parallel lines of L4 L6
  measures "d26" distance of point (30, 5) point (30, 15)
  measures "d27" distance from line of L6 point (30, 15)
  measures "d28" distance of point (20, 15) point (30, 15)
  measures "d29" distance from line of L5 point (30, 15)
  measures "d30" diameter of A0
  measures "d33" distance of A0.centre A1.centre
  measures "d36" distance of A0.centre A2.centre
extrude "Extrusion2" add sketch "Sketch2" along normal blind 7
chamfer "Chamfer1" distance 12.4999 distance2 2 1 edges at (55.5235, 0.9125, 2.5) measured on face at (55.5235, 1.4125, 2.5)
chamfer "Chamfer2" distance 14 distance2 2 2 edges at (55.5235, 7.1625, 0) (55.5235, -2.8375, 0) measured on face at (55.5235, 7.1625, -0.5) measured on face at (55.5235, -2.8375, -0.5)